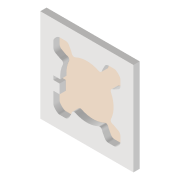
# Autodesk Inventor part: Soporte Cilindro Cortadora
Saved by Autodesk Inventor 2021 (Build 250183000, 183)
## iProperties
Created: 2021-08-10
Part Number: Soporte Cilindro Cortadora
Material: Generic
Document SubType Name: Modeling
Designer: maaro
Density: 1 g/cm^3
Appearance: Default
Author: maaro
Autodesk Inventor part; units mm, degrees
ref_plane "YZ Plane" through (0, 0, 0) normal (1, 0, 0) x (0, 1, 0)
ref_plane "XZ Plane" through (0, 0, 0) normal (0, 1, 0) x (-1, 0, 0)
ref_plane "XY Plane" through (0, 0, 0) normal (0, 0, 1) x (1, 0, 0)
ref_plane "Work Plane1" through (0, 0, 0) normal (0, 0, 1) x (1, 0, 0)
sketch "Sketch1" plane through (0, 0, 0) normal (0, 0, 1) x (1, 0, 0)
  circle A0 centre (0, 0) radius 8
  arc A1 (-21.8566, 27) -> (-23.5705, 26.52) centre (-21.8566, 23.7) ccw
  line L0 (-21.8566, 27) -> (-17.3137, 27)
  arc A2 (-14.4021, 25.2532) -> (-17.3137, 27) centre (-17.3137, 23.7) ccw
  line L1 (-14.4021, 25.2532) -> (-12.8239, 22.2947)
  arc A3 (-12.2013, 20.6664) -> (-12.8239, 22.2947) centre (-19, 19) ccw
  arc A4 (-12.2013, 20.6664) -> (-9.3857, 19.3432) centre (-10.2588, 21.1426) ccw
  arc A5 (9.3857, 19.3432) -> (-9.3857, 19.3432) centre (0, 0) ccw
  arc A6 (9.3857, 19.3432) -> (12.2013, 20.6664) centre (10.2588, 21.1426) ccw
  arc A7 (12.8239, 22.2947) -> (12.2013, 20.6664) centre (19, 19) ccw
  line L2 (12.8239, 22.2947) -> (14.4021, 25.2532)
  arc A8 (17.3137, 27) -> (14.4021, 25.2532) centre (17.3137, 23.7) ccw
  line L3 (17.3137, 27) -> (21.8566, 27)
  arc A9 (23.5705, 26.52) -> (21.8566, 27) centre (21.8566, 23.7) ccw
  arc A10 (26.52, 23.5705) -> (23.5705, 26.52) centre (19, 19) ccw
  arc A11 (27, 21.8566) -> (26.52, 23.5705) centre (23.7, 21.8566) ccw
  line L4 (27, 21.8566) -> (27, 17.3137)
  arc A12 (25.2532, 14.4021) -> (27, 17.3137) centre (23.7, 17.3137) ccw
  line L5 (25.2532, 14.4021) -> (22.2947, 12.8239)
  arc A13 (20.6664, 12.2013) -> (22.2947, 12.8239) centre (19, 19) ccw
  arc A14 (20.6664, 12.2013) -> (19.3432, 9.3857) centre (21.1426, 10.2588) ccw
  arc A15 (19.3432, -9.3857) -> (19.3432, 9.3857) centre (0, 0) ccw
  arc A16 (19.3432, -9.3857) -> (20.6664, -12.2013) centre (21.1426, -10.2588) ccw
  arc A17 (22.2947, -12.8239) -> (20.6664, -12.2013) centre (19, -19) ccw
  line L6 (22.2947, -12.8239) -> (25.2532, -14.4021)
  arc A18 (27, -17.3137) -> (25.2532, -14.4021) centre (23.7, -17.3137) ccw
  line L7 (27, -17.3137) -> (27, -21.8566)
  arc A19 (26.52, -23.5705) -> (27, -21.8566) centre (23.7, -21.8566) ccw
  arc A20 (23.5705, -26.52) -> (26.52, -23.5705) centre (19, -19) ccw
  arc A21 (21.8566, -27) -> (23.5705, -26.52) centre (21.8566, -23.7) ccw
  line L8 (21.8566, -27) -> (17.3137, -27)
  arc A22 (14.4021, -25.2532) -> (17.3137, -27) centre (17.3137, -23.7) ccw
  line L9 (14.4021, -25.2532) -> (12.8239, -22.2947)
  arc A23 (12.2013, -20.6664) -> (12.8239, -22.2947) centre (19, -19) ccw
  arc A24 (12.2013, -20.6664) -> (9.3857, -19.3432) centre (10.2588, -21.1426) ccw
  arc A25 (-9.3857, -19.3432) -> (9.3857, -19.3432) centre (0, 0) ccw
  arc A26 (-9.3857, -19.3432) -> (-12.2013, -20.6664) centre (-10.2588, -21.1426) ccw
  arc A27 (-12.8239, -22.2947) -> (-12.2013, -20.6664) centre (-19, -19) ccw
  line L10 (-12.8239, -22.2947) -> (-14.4021, -25.2532)
  arc A28 (-17.3137, -27) -> (-14.4021, -25.2532) centre (-17.3137, -23.7) ccw
  line L11 (-17.3137, -27) -> (-21.8566, -27)
  arc A29 (-23.5705, -26.52) -> (-21.8566, -27) centre (-21.8566, -23.7) ccw
  arc A30 (-26.52, -23.5705) -> (-23.5705, -26.52) centre (-19, -19) ccw
  arc A31 (-27, -21.8566) -> (-26.52, -23.5705) centre (-23.7, -21.8566) ccw
  line L12 (-27, -21.8566) -> (-27, -12.7696)
  line L13 (-27, -12.7696) -> (-22, -12.7696)
  line L14 (-22, -12.7696) -> (-22, -5.2304)
  line L15 (-22, -5.2304) -> (-27, -5.2304)
  line L16 (-27, -5.2304) -> (-27, -2)
  line L17 (-27, -2) -> (-21.4068, -2)
  arc A32 (-19.3432, 9.3857) -> (-21.4068, -2) centre (0, 0) ccw
  arc A33 (-19.3432, 9.3857) -> (-20.6664, 12.2013) centre (-21.1426, 10.2588) ccw
  arc A34 (-22.2947, 12.8239) -> (-20.6664, 12.2013) centre (-19, 19) ccw
  line L18 (-22.2947, 12.8239) -> (-25.2532, 14.4021)
  arc A35 (-27, 17.3137) -> (-25.2532, 14.4021) centre (-23.7, 17.3137) ccw
  line L19 (-27, 17.3137) -> (-27, 21.8566)
  arc A36 (-26.52, 23.5705) -> (-27, 21.8566) centre (-23.7, 21.8566) ccw
  arc A37 (-23.5705, 26.52) -> (-26.52, 23.5705) centre (-19, 19) ccw
  line L20 (42.5, 37.5) -> (42.5, -37.5)
  line L21 (42.5, -37.5) -> (37.5, -37.5)
  line L22 (37.5, -37.5) -> (37.5, 37.5)
  line L23 (37.5, 37.5) -> (42.5, 37.5)
  line L24 (-42.5, -37.5) -> (-42.5, 37.5)
  line L25 (-42.5, 37.5) -> (-37.5, 37.5)
  line L26 (-37.5, 37.5) -> (-37.5, -37.5)
  line L27 (-37.5, -37.5) -> (-42.5, -37.5)
  line L28 (-37.5, -37.5) -> (37.5, -37.5)
  line L29 (-37.5, 37.5) -> (37.5, 37.5)
  point P0 (0, 0)
  constraints: 74 point on circle, 60 end point, 38 centre point, 12 horizontal, 10 vertical, 1 parallel, 148 other
extrude "Extrusion1" add sketch "Sketch1" along normal blind 5 contours L22 L28 L26 L29
body "Solid1"
